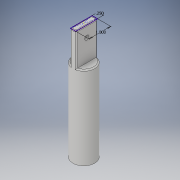
# Autodesk Inventor part: 2016.07.14 magnetic height guide
Saved by Autodesk Inventor 2017 (Build 210142000, 142)
## iProperties
Created: 2016-06-13
Part Number: 2016.07.14 magnetic height guide
Material: Generic
Document SubType Name: Modeling
Designer: Darien Morrow
Density: 1 g/cm^3
Appearance: Default
Author: Darien Morrow
Autodesk Inventor part; units mm, degrees
ref_plane "YZ Plane" through (0, 0, 0) normal (1, 0, 0) x (0, 1, 0)
ref_plane "XZ Plane" through (0, 0, 0) normal (0, 1, 0) x (-1, 0, 0)
ref_plane "XY Plane" through (0, 0, 0) normal (0, 0, 1) x (1, 0, 0)
sketch "Sketch1" plane through (0, 0, 0) normal (0, 0, 1) x (1, 0, 0)
  line L0 (0, 0) -> (12.7, 0)
  line L1 (12.7, 0) -> (12.7, 134.874)
  line L2 (12.7, 134.874) -> (0, 134.874)
  line L3 (0, 134.874) -> (0, 0)
  line L4 (0, 0) -> (2.54, 0)
  line L5 (2.54, 0) -> (2.54, -12.7)
  line L6 (2.54, -12.7) -> (0, -12.7)
  line L7 (0, -12.7) -> (0, 0)
  dimension "d0" = 12.7
  dimension "d1" = 134.874
  dimension "d2" = 12.7
  dimension "d3" = 2.54
  constraints: 16 end point, 4 parallel, 2 horizontal, 2 perpendicular
  measures "d0" distance between parallel lines of L1 L3
  measures "d1" distance between parallel lines of L0 L2
  measures "d2" distance between parallel lines of L6 L0
  measures "d3" distance between parallel lines of L5 L7
revolve "Revolution1" add sketch "Sketch1" angle 360 about axis through (0, 134.874, 0) along (0, -1, 0)
sketch "Sketch4" plane through (0, 134.874, 0) normal (0, 1, 0) x (1, 0, 0)
  line L0 (3.175, -12.7) -> (3.175, 12.7)
  line L1 (3.175, 12.7) -> (-3.175, 12.7)
  line L2 (-3.175, 12.7) -> (-3.175, -12.7)
  line L3 (-3.175, -12.7) -> (3.175, -12.7)
  line L4 (3.175, -12.7) -> (-3.175, 12.7) construction
  line L5 (3.175, 12.7) -> (-3.175, -12.7) construction
  point P0 (0, 0)
  dimension "d24" = 6.35
  dimension "d25" = 25.4
  constraints: 12 end point, 2 midpoint, 2 parallel, 1 perpendicular, 1 vertical
  measures "d24" distance between parallel lines of L0 L2
  measures "d25" distance between parallel lines of L1 L3
sketch "Sketch5" plane through (0, 134.874, 0) normal (0, 1, 0) x (1, 0, 0)
  line L0 (-3.2918, -12.7) -> (-12.7, -12.7)
  line L1 (-12.7, -12.7) -> (-12.7, 12.7)
  line L2 (-12.7, 12.7) -> (-3.2918, 12.7)
  line L3 (-3.2918, 12.7) -> (-3.2918, -12.7)
  line L4 (3.4651, -12.7) -> (12.7, -12.7)
  line L5 (12.7, -12.7) -> (12.7, 12.7)
  line L6 (12.7, 12.7) -> (3.4651, 12.7)
  line L7 (3.4651, 12.7) -> (3.4651, -12.7)
  point P0 (0, 0)
  constraints: 16 end point, 4 parallel, 2 horizontal, 2 perpendicular, 2 point on line
extrude "Extrusion2" cut sketch "Sketch5" against normal blind 38.1
sketch "Sketch6" plane through (3.4651, 134.874, 12.2181) normal (1, 0, 0) x (0, 0, -1)
  line L0 (-0.4819, -134.874) -> (24.9181, -134.874) projected
  line L1 (24.4841, 0) -> (-0.0478, 0) projected
  point P0 (12.2181, -134.874)
  point P1 (12.2181, -12.7)
  dimension "d39" = 12.7
  measures "d39" distance from line of L1 point (12.218, -12.7)
hole "Hole2" at (3.4651, 122.174, 0) direction (-1, 0, 0) diameter 5.08 end through all
chamfer "Chamfer3" distance 1.27 angle 45 12 edges at (10.1316, 96.774, -7.6578) (10.1316, 96.774, 7.6578) (3.4651, 115.824, -12.2181) (3.4651, 115.824, 12.2181) (3.4651, 134.874, 0) (0.0899, 134.874, -12.6997) (0.0899, 134.874, 12.6997) (-3.2918, 134.874, 0) (-3.2918, 115.824, -12.266) (-3.2918, 115.824, 12.266) (-12.7, 96.774, 0) (-2.54, -12.7, 0)
sketch "Sketch7" plane through (0, -12.7, 0) normal (0, -1, 0) x (1, 0, 0)
  circle A0 centre (0, 0) radius 2.54 projected
  circle A1 centre (0, 0) radius 2.54
  point P0 (0, 0)
  constraints: 1 centre point, 1 coincident
extrude "Extrusion3" cut sketch "Sketch7" against normal blind 12.7
sketch "Sketch8" plane through (0, 0, 0) normal (0, -1, 0) x (1, 0, 0)
  point P0 (0, 0)
  point P1 (0, 0)
  constraints: 1 coincident
hole "Hole3" at (0, 0, 0) direction (0, 1, 0) diameter 4.9784 depth 19.05 tip angle 118 thread size "1/4-20 UNC" class "2B" standard "ANSI Unified Screw Threads"
body "Solid1"
